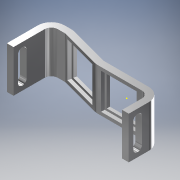
# Autodesk Inventor part: thumbkey_plate
Saved by Autodesk Inventor 2018 (Build 220112000, 112)
## iProperties
Created: 2018-04-07
Part Number: thumbkey_plate
Material: アルミニウム 6061
Document SubType Name: Sheet Metal
Designer: NaMACHAN
Density: 2.7 g/cm^3
Sheet Metal Rule: Default_mm
Appearance: アルミニウム - フラット
Flat Pattern Width: 1.9 cm
Flat Pattern Length: 8.01238 cm
Flat Pattern Area: 15.2235 cm^2
Sheet Metal Width: 19.000 mm
Sheet Metal Length: 80.124 mm
Sheet Metal Area: 1522.352 mm^2
Author: NaMACHAN
Autodesk Inventor part; units mm, degrees
ref_plane "YZ Plane" through (0, 0, 0) normal (1, 0, 0) x (0, 1, 0)
ref_plane "XZ Plane" through (0, 0, 0) normal (0, 1, 0) x (-1, 0, 0)
ref_plane "XY Plane" through (0, 0, 0) normal (0, 0, 1) x (1, 0, 0)
sketch "スケッチ1" plane through (0, 0, 0) normal (0, 1, 0) x (-1, 0, 0)
  line L0 (-10, -9.5) -> (10, -9.5)
  line L1 (10, -9.5) -> (10, 9.5)
  line L2 (10, 9.5) -> (-10, 9.5)
  line L3 (-10, 9.5) -> (-10, -9.5)
  line L4 (-10, -9.5) -> (10, 9.5) construction
  line L5 (10, -9.5) -> (-10, 9.5) construction
  point P0 (0, 0)
  dimension "d0" = 20
  dimension "d1" = 19
  measures "d0" distance of L2.end L1.end
  measures "d1" distance of L1.end L0.end
extrude "プレート1" add sketch "スケッチ1" along normal blind 3
sketch "スケッチ5" plane through (0, 3, 0) normal (0, 1, 0) x (1, 0, 0)
  point P0 (0, 0)
sketch "スケッチ6" plane through (-10.7765, 3.1022, 9.5) normal (-0.258819, -0.9659258, 0) x (0.9659258, -0.258819, 0)
  line L0 (0, -19) -> (0, 0)
  line L1 (0, 0) -> (-18.2101, 0)
  line L2 (-18.2101, 0) -> (-18.2101, -19)
  line L3 (-18.2101, -19) -> (0, -19)
  constraints: 6 end point, 1 horizontal, 1 perpendicular, 1 vertical
edge flange "フランジ3" height 19 angle 15 thickness 3 bend radius 3 thickness toward (-0.258819, -0.9659258, 0) relief tear relief width 3 relief depth 1.5 edges at (-10, 3, 0) wall of the first edge with corners at (-10.7765, 3.1022, -9.5) (-10.7765, 3.1022, 9.5) (-28.366, 7.8153, 9.5) (-28.366, 7.8153, -9.5)
bend "曲げ3"
corner "コーナー3"
sketch "スケッチ7" plane through (-29.919, 5.0198, 9.5) normal (0, 1, 0) x (1, 0, 0)
  line L0 (0, -19) -> (0, 0)
  line L1 (0, 0) -> (-3.0801, 0)
  line L2 (-3.0801, 0) -> (-3.0801, -19)
  line L3 (-3.0801, -19) -> (0, -19)
  constraints: 6 end point, 1 horizontal, 1 perpendicular, 1 vertical
edge flange "フランジ4" height 3.87 angle -15 thickness 3 bend radius 3 thickness toward (0, 1, 0) relief tear relief width 3 relief depth 1.5 edges at (-28.366, 7.8153, 0) wall of the first edge with corners at (-29.919, 5.0198, -9.5) (-29.919, 5.0198, 9.5) (-32.999, 5.0198, 9.5) (-32.999, 5.0198, -9.5)
bend "曲げ4"
corner "コーナー4"
sketch "スケッチ8" plane through (13, -3, -9.5) normal (1, 0, 0) x (0, -1, 0)
  line L0 (0, 19) -> (0, 0)
  line L1 (0, 0) -> (9, 0)
  line L2 (9, 0) -> (9, 19)
  line L3 (9, 19) -> (0, 19)
  constraints: 6 end point, 1 horizontal, 1 perpendicular, 1 vertical
edge flange "フランジ5" height 15 angle -90 thickness 3 bend radius 3 thickness toward (1, 0, 0) relief tear relief width 3 relief depth 1.5 edges at (10, 3, 0) wall of the first edge with corners at (13, -3, 9.5) (13, -3, -9.5) (13, -12, -9.5) (13, -12, 9.5)
bend "曲げ5"
corner "コーナー5"
sketch "スケッチ9" plane through (-35.999, 2.0198, 9.5) normal (-1, 0, 0) x (0, 1, 0)
  line L0 (0, -19) -> (0, 0)
  line L1 (0, 0) -> (-14, 0)
  line L2 (-14, 0) -> (-14, -19)
  line L3 (-14, -19) -> (0, -19)
  constraints: 8 end point
edge flange "フランジ6" height 20 angle -90 thickness 3 bend radius 3 thickness toward (-1, 0, 0) relief tear relief width 3 relief depth 1.5 edges at (-32.999, 8.0198, 0) wall of the first edge with corners at (-35.999, 2.0198, -9.5) (-35.999, 2.0198, 9.5) (-35.999, -11.9802, 9.5) (-35.999, -11.9802, -9.5)
bend "曲げ6"
corner "コーナー6"
sketch "スケッチ14" plane through (16, -12, 9.5) normal (1, 0, 0) x (0, 0, -1)
  line L0 (4, 6) -> (15, 6)
  arc A0 (15, 2) -> (15, 6) centre (15, 4) ccw
  line L1 (15, 2) -> (4, 2)
  arc A1 (4, 6) -> (4, 2) centre (4, 4) ccw
  line L2 (19, 9) -> (19, 0) projected
  line L3 (0, 9) -> (0, 0) projected
  line L4 (0, 0) -> (19, 0) projected
  point P0 (9.5, 12)
  dimension "d86" = 2
  dimension "d87" = 4
  dimension "d88" = 4
  dimension "d89" = 4
  constraints: 4 end point, 4 point on circle, 4 tangent, 2 centre point, 1 horizontal, 1 parallel
  measures "d86" radius of A1
  measures "d87" distance from line of L2 A0.centre
  measures "d88" distance from line of L3 A1.centre
  measures "d89" distance from line of L4 A1.centre
extrude "押し出し6" cut sketch "スケッチ14" against normal blind 100
sketch "スケッチ15" plane through (0, 0, 0) normal (0, -1, 0) x (1, 0, 0)
  line L0 (7.5, -8) -> (-8.5, -8)
  line L1 (-8.5, -8) -> (-8.5, 8)
  line L2 (-8.5, 8) -> (7.5, 8)
  line L3 (7.5, 8) -> (7.5, -8)
  line L4 (7.5, -8) -> (-8.5, 8) construction
  line L5 (-8.5, -8) -> (7.5, 8) construction
  line L6 (-10, -9.5) -> (-10, 9.5) projected
  point P0 (0, 0)
  point P1 (-0.5, 0)
  point P2 (-0.5, 0)
  dimension "d92" = 16
  dimension "d93" = 16
  dimension "d94" = 9.5
  constraints: 12 end point, 3 midpoint, 2 parallel, 1 horizontal, 1 horizontal alignment, 1 perpendicular
  measures "d92" distance of L1.end L2.end
  measures "d93" distance of L0.end L1.end
  measures "d94" distance from line of L6 point (-0.5, 0)
extrude "押し出し7" cut sketch "スケッチ15" against normal blind 1.6
sketch "スケッチ16" plane through (0, 1.6, 0) normal (0, -1, 0) x (1, 0, 0)
  line L0 (-7.5, -7) -> (6.5, -7)
  line L1 (6.5, -7) -> (6.5, 7)
  line L2 (6.5, 7) -> (-7.5, 7)
  line L3 (-7.5, 7) -> (-7.5, -7)
  line L4 (-7.5, -7) -> (6.5, 7) construction
  line L5 (6.5, -7) -> (-7.5, 7) construction
  line L6 (7.5, -8) -> (-8.5, -8) projected
  line L7 (7.5, 8) -> (7.5, -8) projected
  point P0 (0, 0)
  point P1 (-0.5, 0)
  point P2 (-0.5, 0)
  point P3 (-0.5, -8)
  point P4 (7.5, 0)
  dimension "d97" = 14
  dimension "d98" = 14
  constraints: 12 end point, 5 midpoint, 2 parallel, 1 horizontal, 1 horizontal alignment, 1 perpendicular, 1 vertical alignment
  measures "d97" distance of L2.end L1.end
  measures "d98" distance of L1.end L0.end
extrude "押し出し8" cut sketch "スケッチ16" against normal blind 1.4
sketch "スケッチ17" plane through (-11.5529, 0.2044, -9.5) normal (-0.258819, -0.9659258, 0) x (0.9659258, -0.258819, 0)
  line L0 (-17.5, 1.5) -> (-1.5, 1.5)
  line L1 (-1.5, 1.5) -> (-1.5, 17.5)
  line L2 (-1.5, 17.5) -> (-17.5, 17.5)
  line L3 (-17.5, 17.5) -> (-17.5, 1.5)
  line L4 (-17.5, 1.5) -> (-1.5, 17.5) construction
  line L5 (-1.5, 1.5) -> (-17.5, 17.5) construction
  line L6 (0, 0) -> (0, 19) projected
  point P0 (11.2122, 9.5)
  point P1 (-9.5, 9.5)
  point P2 (-9.5, 9.5)
  point P3 (0, 9.5)
  dimension "d101" = 16
  dimension "d102" = 16
  dimension "d103" = 9.5
  constraints: 12 end point, 4 midpoint, 2 parallel, 1 horizontal, 1 horizontal alignment, 1 perpendicular
  measures "d101" distance of L2.end L1.end
  measures "d102" distance of L1.end L0.end
  measures "d103" distance from line of L6 point (-9.5, 9.5)
extrude "押し出し9" cut sketch "スケッチ17" against normal blind 1.6
sketch "スケッチ18" plane through (-11.1388, 1.7499, -9.5) normal (-0.258819, -0.9659258, 0) x (0.9659258, -0.258819, 0)
  line L0 (-16.5, 2.5) -> (-2.5, 2.5)
  line L1 (-2.5, 2.5) -> (-2.5, 16.5)
  line L2 (-2.5, 16.5) -> (-16.5, 16.5)
  line L3 (-16.5, 16.5) -> (-16.5, 2.5)
  line L4 (-16.5, 2.5) -> (-2.5, 16.5) construction
  line L5 (-2.5, 2.5) -> (-16.5, 16.5) construction
  line L6 (-1.5, 17.5) -> (-1.5, 1.5) projected
  line L7 (-18.2101, 0) -> (0, 0) projected
  line L8 (-1.5, 1.5) -> (-17.5, 1.5) projected
  point P0 (11.2122, 9.5)
  point P1 (-9.5, 9.5)
  point P2 (-9.5, 9.5)
  point P3 (-1.5, 9.5)
  point P4 (-9.5, 9.5)
  point P5 (-9.5, 16.5)
  point P6 (-9.105, 0)
  point P7 (-9.5, 1.5)
  dimension "d106" = 14
  dimension "d107" = 14
  constraints: 12 end point, 8 midpoint, 2 parallel, 1 horizontal, 1 horizontal alignment, 1 perpendicular, 1 vertical alignment
  measures "d106" distance of L2.end L1.end
  measures "d107" distance of L1.end L0.end
extrude "押し出し10" cut sketch "スケッチ18" against normal blind 1.4
equation "\"d2\" = Thickness"
equation "\"d29\" = BendReliefWidth"
equation "\"d30\" = BendReliefDepth"
equation "\"d31\" = MinimumRemnant"
equation "\"d32\" = TransitionRadius"
equation "\"d35\" = BendRadius"
equation "\"d36\" = CornerReliefSize"
equation "\"d37\" = GapSize"
equation "\"d38\" = JacobiRadiusSize"
equation "\"d39\" = BendReliefWidth"
equation "\"d40\" = BendReliefDepth"
equation "\"d41\" = MinimumRemnant"
equation "\"d42\" = TransitionRadius"
equation "\"d45\" = BendRadius"
equation "\"d46\" = CornerReliefSize"
equation "\"d47\" = GapSize"
equation "\"d48\" = JacobiRadiusSize"
equation "\"d49\" = BendReliefWidth"
equation "\"d50\" = BendReliefDepth"
equation "\"d51\" = MinimumRemnant"
equation "\"d52\" = TransitionRadius"
equation "\"d55\" = BendRadius"
equation "\"d56\" = CornerReliefSize"
equation "\"d57\" = GapSize"
equation "\"d58\" = JacobiRadiusSize"
equation "\"d59\" = BendReliefWidth"
equation "\"d60\" = BendReliefDepth"
equation "\"d61\" = MinimumRemnant"
equation "\"d62\" = TransitionRadius"
equation "\"d65\" = BendRadius"
equation "\"d66\" = CornerReliefSize"
equation "\"d67\" = GapSize"
equation "\"d68\" = JacobiRadiusSize"
equation "\"BendRadius\" = Thickness"
equation "\"BendReliefWidth\" = Thickness"
equation "\"BendReliefDepth\" = 0.5 * Thickness"
equation "\"CornerReliefSize\" = 4 * Thickness"
equation "\"MinimumRemnant\" = 2 * Thickness"
equation "\"TransitionRadius\" = BendRadius"
equation "\"JacobiRadiusSize\" = BendRadius"
equation "\"GapSize\" = Thickness"
equation "\"Thickness\" = 3"
